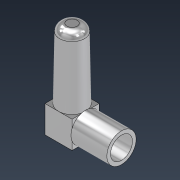
# Autodesk Inventor part: Antenne-Klein
Saved by Autodesk Inventor 2022.1 (Build 261234020, 234B)
## iProperties
Created: 2015-09-02
Part Number: Antenne-Klein
Material: Aluminium 6061
Document SubType Name: Modeling
Designer: rYan
Density: 2.7 g/cm^3
Appearance: Aluminium - flach
Mass: 3.64939 g
Surface Area: 11.5991 cm^2
Volume: 1.35163 cm^3
Author: rYan
Autodesk Inventor part; units mm, degrees
ref_plane "YZ Plane" through (0, 0, 0) normal (1, 0, 0) x (0, 1, 0)
ref_plane "XZ Plane" through (0, 0, 0) normal (0, 1, 0) x (-1, 0, 0)
ref_plane "XY Plane" through (0, 0, 0) normal (0, 0, 1) x (1, 0, 0)
sketch "Skizze1" plane through (0, 0, 0) normal (0, 0, 1) x (1, 0, 0)
  line L0 (-3.7, 3.7) -> (3.7, 3.7)
  line L1 (3.7, 3.7) -> (3.7, -3.7)
  line L2 (3.7, -3.7) -> (-3.7, -3.7)
  line L3 (-3.7, -3.7) -> (-3.7, 3.7)
  line L4 (0, 5.18) -> (0, -5.18) projected
  line L5 (-5.18, 0) -> (5.18, 0) projected
  point P0 (0, 0)
  dimension "d0" = 7.4
  dimension "d1" = 7.4
  constraints: 8 end point, 2 parallel, 1 horizontal, 1 perpendicular, 2 other
  measures "d0" distance of L0.start L0.end
  measures "d1" distance of L0.end L1.end
extrude "Extrusion1" add sketch "Skizze1" against normal blind 7.4
sketch "Skizze2" plane through (0, 0, 0) normal (0, 0, 1) x (1, 0, 0)
  circle A0 centre (0, 0) radius 3.7
  dimension "d4" = 7.4
  constraints: 1 centre point, 1 coincident
  measures "d4" diameter of A0
extrude "Extrusion2" add sketch "Skizze2" along normal blind 19 draft -1
fillet "Rundung1" radius 2 1 edges at (-3.3684, 0, 19)
sketch "Skizze3" plane through (3.7, -3.7, -7.4) normal (1, 0, 0) x (0, 0, -1)
  line L0 (-7.4, 7.4) -> (-7.4, 3.7) projected
  line L1 (-7.4, 3.7) -> (-7.4, 0) projected
  line L2 (-7.4, 0) -> (0, 0) projected
  line L3 (0, 7.4) -> (0, 0) projected
  line L4 (-7.4, 7.4) -> (0, 7.4) projected
  line L5 (-7.4, 3.7) -> (0, 3.7) construction
  line L6 (0, 7.4) -> (0, 0) construction
  line L7 (-7.4, 0) -> (0, 0) construction
  line L8 (-3.7, 0) -> (-3.7, 7.4) construction
  line L9 (-7.4, 7.4) -> (0, 7.4) construction
  circle A0 centre (-3.7, 3.7) radius 4
  circle A1 centre (-3.7, 3.7) radius 3
  dimension "d8" = 8
  dimension "d9" = 6
  constraints: 4 end point, 4 midpoint, 2 centre point, 1 coincident
  measures "d8" diameter of A0
  measures "d9" diameter of A1
extrude "Extrusion3" add sketch "Skizze3" along normal blind 9.8 contours A0 L4 L3 L2 L1 L0 | L0 L1 A0 | A0 L4 | L2 A0 | A0 L3
